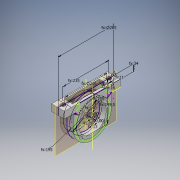
# Autodesk Inventor part: корпус подшипника1
Saved by Autodesk Inventor 2018.3 (Build 223284000, 284)
## iProperties
Created: 2018-05-09
Part Number: корпус подшипника1
Material: Типовые
Document SubType Name: Modeling
Designer: kriku
Density: 1 g/cm^3
Appearance: По умолчанию
Mass: 860.772 g
Surface Area: 1208.71 cm^2
Volume: 860.772 cm^3
Author: kriku
Autodesk Inventor part; units mm, degrees
ref_plane "XZ Plane" through (0, 0, 0) normal (0, 1, 0) x (-1, 0, 0)
ref_plane "XY Plane" through (0, 0, 0) normal (0, 0, 1) x (1, 0, 0)
sketch "Эскиз1" plane through (0, 0, 0) normal (1, 0, 0) x (0, 1, 0)
  circle A0 centre (0, 0) radius 70
  circle A1 centre (0, 0) radius 82.5
  arc A2 (80.4212, 18.894) -> (80.3103, 18.8815) centre (82.3009, 1.7165) ccw
  circle A3 centre (0, 0) radius 97.5
  line L0 (142.5, 102) -> (108, 102)
  line L1 (0, -132.6) -> (0, 165.6) projected
  line L2 (142.5, 102) -> (142.5, 68)
  line L3 (108, 102) -> (108, 101.5)
  line L4 (108, 101.5) -> (0, 101.5)
  line L5 (-142.5, 102) -> (-108, 102)
  line L6 (-142.5, 102) -> (-142.5, 68)
  line L7 (-108, 102) -> (-108, 101.5)
  line L8 (-108, 101.5) -> (0, 101.5)
  arc A4 (11.7449, -38.2368) -> (27.2385, -29.2927) centre (0, 0) ccw
  arc A5 (-27.2416, -29.2898) -> (-11.749, -38.2356) centre (0, 0) ccw
  line L9 (-142.5, 68) -> (-69.8731, 68)
  line L10 (97.5, 0) -> (97.5, 68)
  line L11 (142.5, 68) -> (69.8731, 68)
  line L12 (-97.5, 0) -> (-97.5, 68)
  line L13 (117.5, 43) -> (117.5, 123)
  line L14 (-117.5, 43) -> (-117.5, 123)
  line L15 (133.5, 68) -> (117.5, 68)
  line L16 (117.5, 68) -> (117.5, 69)
  line L17 (117.5, 69) -> (133.5, 69)
  line L18 (133.5, 69) -> (133.5, 68)
  line L19 (128.5, 69) -> (117.5, 69)
  line L20 (117.5, 69) -> (117.5, 85)
  line L21 (128.5, 102) -> (128.5, 69)
  line L22 (133.5, 102) -> (117.5, 102)
  line L23 (117.5, 69) -> (101.5, 69)
  line L24 (101.5, 69) -> (101.5, 68)
  line L25 (106.5, 101.5) -> (106.5, 69)
  line L26 (-108, 102) -> (-108, 101.5)
  line L27 (-133.5, 68) -> (-117.5, 68)
  line L28 (-117.5, 68) -> (-117.5, 69)
  line L29 (-117.5, 69) -> (-133.5, 69)
  line L30 (-133.5, 69) -> (-133.5, 68)
  line L31 (-128.5, 69) -> (-117.5, 69)
  line L32 (-117.5, 69) -> (-117.5, 85)
  line L33 (-128.5, 102) -> (-128.5, 69)
  line L34 (-133.5, 102) -> (-117.5, 102)
  line L35 (-101.5, 69) -> (-101.5, 68)
  line L36 (-117.5, 69) -> (-101.5, 69)
  line L37 (-106.5, 101.5) -> (-106.5, 69)
  line L38 (117.5, 68) -> (117.5, 102)
  line L39 (-117.5, 68) -> (-117.5, 102)
  line L40 (0, 0) -> (69.6414, -69.6414)
  circle A6 centre (58.3363, -58.3363) radius 6.5
  circle A7 centre (58.3363, 58.3363) radius 6.5
  circle A8 centre (-58.3363, 58.3363) radius 6.5
  circle A9 centre (-58.3363, -58.3363) radius 6.5
  arc A10 (69.8731, 68) -> (-69.8731, 68) centre (0, 0) ccw
  line L41 (97.5, 68) -> (69.8731, 68)
  line L42 (-69.8731, 68) -> (-97.5, 68)
  line L43 (128.5, 69) -> (128.5, 102)
  line L44 (89, 68) -> (89, 101.5)
  arc A11 (83.0142, 68) -> (79.5188, 56.4182) centre (116.097, 51.6972) ccw
  arc A12 (79.5188, 56.4182) -> (62.6803, 74.6822) centre (0, 0) ccw
  line L45 (83.0142, 68) -> (83.0142, 84.568)
  line L46 (83.0142, 84.568) -> (89, 84.568)
  arc A13 (79.5188, 56.4182) -> (62.6803, 74.6822) centre (0, 0) ccw
  line L47 (-101.5, 69) -> (-101.5, 68)
  line L48 (-97.5, 68) -> (-69.8731, 68)
  arc A14 (-79.5188, 56.4182) -> (-83.0142, 68) centre (-116.097, 51.6972) ccw
  arc A15 (-62.6803, 74.6822) -> (-79.5188, 56.4182) centre (0, 0) ccw
  line L49 (-83.0142, 68) -> (-83.0142, 84.568)
  line L50 (-83.0142, 84.568) -> (-89, 84.568)
  arc A16 (-62.6803, 74.6822) -> (-79.5188, 56.4182) centre (0, 0) ccw
  line L51 (0, 97.5) -> (0, 101.5)
  line L52 (0, 101.5) -> (89, 101.5)
  line L53 (89, 101.5) -> (89, 84.568)
  arc A17 (62.6803, 74.6822) -> (0, 97.5) centre (0, 0) ccw
  arc A18 (89, 84.568) -> (47.9908, 67.1054) centre (89, 27.6838) ccw
  arc A19 (47.9908, 67.1054) -> (0, 82.5) centre (0, 0) ccw
  line L54 (79.5188, 56.4182) -> (60.3628, 70.1005)
  line L55 (60.3628, 70.1005) -> (47.9908, 67.1054)
  arc A20 (-47.9908, 67.1054) -> (-89, 84.568) centre (-89, 27.6838) ccw
  line L56 (-79.5188, 56.4182) -> (-59.1498, 66.8423)
  line L57 (-59.1498, 66.8423) -> (-47.9908, 67.1054)
  line L58 (0, 101.5) -> (-89, 101.5)
  line L59 (-89, 101.5) -> (-89, 84.568)
  arc A21 (-47.9908, 67.1054) -> (-89, 84.568) centre (-89, 27.6838) ccw
  arc A22 (0, 82.5) -> (-47.9908, 67.1054) centre (0, 0) ccw
  arc A23 (47.9908, 67.1054) -> (-47.9908, 67.1054) centre (0, 0) ccw
  point P0 (80.4117, 18.4447)
  point P1 (0, -97.5)
  point P2 (128.5, 85)
  point P3 (106.5, 85)
  point P4 (-128.5, 85)
  point P5 (-106.5, 85)
  point P6 (-89, 68)
  dimension "d0" = 140
  dimension "d4" = 165
  dimension "d19" = 195
  dimension "d20" = 199.5
  dimension "d22" = 285
  dimension "d23" = 216
  dimension "d24" = 0.5
  dimension "d46" = 34
  dimension "d64" = 235
  dimension "d65" = 16
  dimension "d66" = 11
  dimension "d67" = 1
  dimension "d70" = 45
  dimension "d71" = 13
  dimension "d74" = 360
  dimension "d84" = 12.5
  constraints: 118 end point, 47 point on circle, 35 symmetric about line, 28 point on line, 24 centre point, 12 coincident, 7 vertical, 6 collinear, 6 horizontal, 5 perpendicular, 4 parallel, 2 tangent, 1 horizontal alignment, 1 vertical alignment, 16 other
  measures "d0" diameter of A0
  measures "d4" diameter of A1
  measures "d19" diameter of A3
  measures "d20" distance from line of L0 A3.start
  measures "d22" diameter of L2 L1
  measures "d23" diameter of L3 L1
  measures "d24" distance between parallel lines of L0 L4
  measures "d46" distance between parallel lines of L0 L11
  measures "d64" distance between parallel lines of L14 L13
  measures "d65" distance between parallel lines of L16 L18
  measures "d66" distance between parallel lines of L20 L21
  measures "d67" distance between parallel lines of L15 L17
  measures "d70" angle of L1 L40
  measures "d71" diameter of A6
  measures "d84" distance between parallel lines of L24 L44
extrude "Выдавливание1" add sketch "Эскиз1" along normal blind 34 and the other way blind 34 contours A0 L1 A1 A7 A6 L40 | A0 L1 A1 A9 A8 | L40 A6 A1 L1 A0 | A6 A1 L40 | L40 A1 A6 | A1 A9 | A1 A7 | A8 A1 picked at (57.6773, -55.9908) picked at (55.9908, -57.6773) picked at (-56.6588, -56.9353) picked at (56.9815, 56.6214) picked at (-56.6588, 56.9353)
extrude "Выдавливание2" add sketch "Эскиз1" along normal blind 34 and the other way blind 34 contours A0 L40 L1 | A0 L1 A1 A7 A6 L40 | L1 A0 | A0 L1 A1 A9 A8 | L40 A6 A1 L1 A0 | A0 L1 L40 | A6 A1 L40 | L40 A1 A6 | A1 A9 | A1 A7 | A8 A1 picked at (57.6773, -55.9908) picked at (55.9908, -57.6773) picked at (-56.6588, -56.9353) picked at (56.9815, 56.6214) picked at (-56.6588, 56.9353)
pattern_circular "Круговой массив1" count 6 over 360 about axis through (0, 0, 0) along (1, 0, 0) of "Выдавливание2"
extrude "Выдавливание3" add sketch "Эскиз1" along normal blind 33 and the other way blind 33 contours A0 L40 L1 | A0 L1 A1 A7 A6 L40 | L1 A0 | A0 L1 A1 A9 A8 | L40 A6 A1 L1 A0 | A0 L1 L40 | L1 A3 A18 A1 | A1 A20 A3 L1 | A6 A1 L40 | L40 A1 A6 | L1 A3 L56 L57 A1 A8 A9 | A1 A6 L40 A3 L1 | L55 L54 A3 L40 A6 A1 A7 | A18 A3 L54 L55 | L57 L56 A3 A20 | L40 A6 A1 | A1 A6 L40 | A9 A1 | A1 A9 | A7 A1 | A1 A7 | A8 A1 | A1 A8 | A11 L11 L10 A3 | A3 L11 A11
extrude "Выдавливание4" add sketch "Эскиз1" along normal blind 33 and the other way blind 33 contours L12 L9 A14 A3 | A14 L9 A3
extrude "Выдавливание7" add sketch "Эскиз1" along normal blind 33 and the other way blind 33 contours A0 L40 L1 | A0 L1 A1 A7 A6 L40 | L1 A0 | A0 L1 A1 A9 A8 | L40 A6 A1 L1 A0 | A0 L1 L40 | L1 A3 A18 A1 | A1 A20 A3 L1 | L1 A3 L56 L57 A1 A8 A9 | A1 A6 L40 A3 L1 | L55 L54 A3 L40 A6 A1 A7 | A18 A3 L54 L55 | L57 L56 A3 A20 | L1 L4 L44 L46 L45 A18 A3 | A3 A20 L49 L50 L59 L8 L1 | A18 L45 L11 A3 | A3 L9 L49 A20 | A18 L44 L11 L45 | L45 L46 A18 | A20 L50 L49 | L49 L9 L35 L36 L37 L8 L59 A20 | L4 L25 L23 L24 L11 L44 | L37 L36 L14 L5 L7 L8 | L9 L14 L36 L35 | L23 L13 L11 L24 | L9 L30 L29 L14 | L17 L18 L11 L13 | L29 L33 L5 L14 | L9 L6 L5 L33 L29 L30 | L21 L0 L2 L11 L18 L17
extrude "Выдавливание8" add sketch "Эскиз1" along normal blind 33 and the other way blind 33 contours L4 L3 L0 L13 L23 L25 | L17 L18 L11 L13 | L13 L0 L21 L17 | L21 L0 L2 L11 L18 L17
revolve "Вращение2" cut sketch "Эскиз1" angle 360 about axis through (0, -117.5, 43) along (0, 0, 1) contours L9 L30 L29 L14 | L29 L33 L5 L14
extrude "Выдавливание9" add sketch "Эскиз1" along normal blind 33 and the other way blind 33 contours A18 L44 L11 L45 | L45 L46 A18 | L4 L25 L23 L24 L11 L44 | L23 L13 L11 L24 | L17 L18 L11 L13
extrude "Выдавливание11" [suppressed]
revolve "Вращение1" cut sketch "Эскиз1" angle 360 about axis through (0, 117.5, 43) along (0, 0, 1) contours L17 L18 L11 L13 | L13 L0 L21 L17
extrude "Выдавливание12" cut sketch "Эскиз1" along normal blind 21 and the other way blind 21 contours L1 A3 A18 A1 | A1 A20 A3 L1 | L1 L4 L44 L46 L45 A18 A3 | A3 A20 L49 L50 L59 L8 L1 | L45 L46 A18 | A20 L50 L49
extrude "Выдавливание13" cut sketch "Эскиз1" along normal through all both and the other way through all contours A6 A1 L40 | L40 A1 A6 | L40 A6 A1 | A1 A6 L40 | A9 A1 | A1 A9 | A7 A1 | A1 A7 | A8 A1 | A1 A8
extrude "Выдавливание14" cut sketch "Эскиз1" along normal through all both and the other way through all contours A0 L40 L1 | L1 A0 | A0 L1 L40
sketch "Эскиз3" plane through (34, 0, 0) normal (1, 0, 0) x (0, 0, -1)
  line L0 (-68, 97.5) -> (-68, 142.5) projected
  line L1 (-68, 97.5) -> (-68, 86.5)
  line L2 (-68, 86.5) -> (-85, 67.5)
  line L3 (-85, 67.5) -> (-101.5, 67.5)
  line L4 (-101.5, 89) -> (-101.5, -89) projected
  line L5 (-101.5, 67.5) -> (-101.5, 0)
  arc A0 (0, 97.5) -> (0, 97.5) centre (0, 0) ccw projected
  line L6 (-68, 97.5) -> (-52.0783, 73.402)
  line L7 (137.4, 0) -> (-141.9, 0) projected
  line L8 (-68, -97.5) -> (-64, -83.0142)
  line L9 (-68, -97.5) -> (-68, -86.5)
  line L10 (-68, -86.5) -> (-85, -67.5)
  line L11 (-85, -67.5) -> (-101.5, -67.5)
  line L12 (-101.5, -67.5) -> (-101.5, 0)
  line L13 (-68, -97.5) -> (-52.0783, -73.402)
  arc A1 (-64, 83.0142) -> (-52.0783, 73.402) centre (-35.394, 106.294) ccw projected
  arc A2 (-52.0783, -73.402) -> (-64, -83.0142) centre (-35.394, -106.294) ccw projected
  arc A3 (-52.0783, 73.402) -> (-52.0783, -73.402) centre (0, 0) ccw
  point P0 (-68, 142.5)
  constraints: 22 end point, 6 symmetric about line, 2 coincident, 2 point on circle, 1 centre point, 1 midpoint, 1 perpendicular, 1 point on line, 1 vertical, 4 other
extrude "Выдавливание15" [suppressed]
extrude "Выдавливание16" [suppressed]
sketch "Эскиз4" plane through (-34, 0, 0) normal (-1, 0, 0) x (0, -1, 0)
  circle A0 centre (-58.3363, -58.3363) radius 6.5 projected
  arc A1 (-66.7759, -48.4482) -> (-58.3363, -58.3363) centre (0, 0) ccw
  arc A2 (-66.7759, -48.4482) -> (-48.4482, -66.7759) centre (-58.3363, -58.3363) ccw
  arc A3 (-58.3363, -58.3363) -> (-48.4482, -66.7759) centre (0, 0) ccw
  arc A4 (-62.7479, -53.5626) -> (-53.5626, -62.7479) centre (-58.3363, -58.3363) ccw
  arc A5 (-53.5626, -62.7479) -> (-48.4482, -66.7759) centre (0, 0) ccw
  arc A6 (-66.7759, -48.4482) -> (-62.7479, -53.5626) centre (0, 0) ccw
  arc A7 (48.4482, -66.7759) -> (58.3363, -58.3363) centre (0, 0) ccw
  arc A8 (48.4482, -66.7759) -> (66.7759, -48.4482) centre (58.3363, -58.3363) ccw
  arc A9 (58.3363, -58.3363) -> (66.7759, -48.4482) centre (0, 0) ccw
  arc A10 (53.5626, -62.7479) -> (62.7479, -53.5626) centre (58.3363, -58.3363) ccw
  arc A11 (62.7479, -53.5626) -> (66.7759, -48.4482) centre (0, 0) ccw
  arc A12 (48.4482, -66.7759) -> (53.5626, -62.7479) centre (0, 0) ccw
  arc A13 (66.7759, 48.4482) -> (58.3363, 58.3363) centre (0, 0) ccw
  arc A14 (66.7759, 48.4482) -> (48.4482, 66.7759) centre (58.3363, 58.3363) ccw
  arc A15 (58.3363, 58.3363) -> (48.4482, 66.7759) centre (0, 0) ccw
  arc A16 (62.7479, 53.5626) -> (53.5626, 62.7479) centre (58.3363, 58.3363) ccw
  arc A17 (53.5626, 62.7479) -> (48.4482, 66.7759) centre (0, 0) ccw
  arc A18 (66.7759, 48.4482) -> (62.7479, 53.5626) centre (0, 0) ccw
  arc A19 (-48.4482, 66.7759) -> (-58.3363, 58.3363) centre (0, 0) ccw
  arc A20 (-48.4482, 66.7759) -> (-66.7759, 48.4482) centre (-58.3363, 58.3363) ccw
  arc A21 (-58.3363, 58.3363) -> (-66.7759, 48.4482) centre (0, 0) ccw
  arc A22 (-53.5626, 62.7479) -> (-62.7479, 53.5626) centre (-58.3363, 58.3363) ccw
  arc A23 (-62.7479, 53.5626) -> (-66.7759, 48.4482) centre (0, 0) ccw
  arc A24 (-48.4482, 66.7759) -> (-53.5626, 62.7479) centre (0, 0) ccw
  arc A25 (-66.7759, -48.4482) -> (-48.4482, -66.7759) centre (0, 0) ccw
  arc A26 (-66.7759, -48.4482) -> (-48.4482, -66.7759) centre (0, 0) ccw
  arc A27 (-66.7759, -48.4482) -> (-48.4482, -66.7759) centre (0, 0) ccw
  arc A28 (-66.7759, -48.4482) -> (-48.4482, -66.7759) centre (-58.3363, -58.3363) ccw
  dimension "d112" = 360
  dimension "d116" = 360
  dimension "d118" = 13
  constraints: 78 point on circle, 28 centre point, 23 coincident, 82 other
  measures "d118" radius of A2
equation "\"d0\" = D"
equation "\"d4\" = D1"
equation "\"d19\" = -2 * H1 + 2 * H_"
equation "\"d20\" = H_"
equation "\"d22\" = L"
equation "\"d23\" = t"
equation "\"d46\" = h_"
equation "\"d64\" = L2"
equation "\"d65\" = 0.5 * d3"
equation "\"d66\" = 0.5 * d1"
equation "\"d71\" = d"
equation "\"d25\" = 0.5 * B"
equation "\"d26\" = 0.5 * B"
equation "\"d34\" = 0.5 * B"
equation "\"d35\" = 0.5 * B"
equation "\"d76\" = 0.5 * B1"
equation "\"d77\" = 0.5 * B1"
equation "\"d80\" = 0.5 * B1"
equation "\"d81\" = 0.5 * B1"
equation "\"d85\" = 0.5 * B1"
equation "\"d86\" = 0.5 * B1"
equation "\"d94\" = 0.5 * B1"
equation "\"d95\" = 0.5 * B"
equation "\"D\" = 140"
equation "\"D1\" = 165"
equation "\"d\" = 13"
equation "\"del\" = 0.12"
equation "\"d1\" = 22"
equation "\"L2\" = 235"
equation "\"B\" = 68"
equation "\"B1\" = 66"
equation "\"L\" = 285"
equation "\"L1\" = 195"
equation "\"t\" = 216"
equation "\"H_\" = 199.5"
equation "\"H1\" = 102"
equation "\"h_\" = 34"
equation "\"d3\" = 32"
